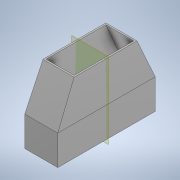
# Autodesk Inventor part: Guía
Saved by Autodesk Inventor 2020.3 (Build 243373000, 373)
## iProperties
Created: 2020-07-24
Part Number: Guía
Material: ABS Plastic
Document SubType Name: Modeling
Designer: juanp
Density: 1.06 g/cm^3
Appearance: Smooth - White
Author: juanp
Autodesk Inventor part; units mm, degrees
ref_plane "YZ Plane" through (0, 0, 0) normal (1, 0, 0) x (0, 1, 0)
ref_plane "XZ Plane" through (0, 0, 0) normal (0, 1, 0) x (-1, 0, 0)
ref_plane "XY Plane" through (0, 0, 0) normal (0, 0, 1) x (1, 0, 0)
sketch "Sketch1" plane through (0, 0, 0) normal (0, 1, 0) x (-1, 0, 0)
  line L0 (0, 0) -> (38, 0)
  line L1 (38, 0) -> (38, 120)
  line L2 (38, 120) -> (0, 120)
  line L3 (0, 120) -> (0, 0)
  line L4 (40, 122) -> (-2, 122)
  line L5 (-2, 122) -> (-2, -2)
  line L6 (-2, -2) -> (40, -2)
  line L7 (40, -2) -> (40, 122)
  line L8 (40, 122) -> (-2, -2) construction
  line L9 (-2, 122) -> (40, -2) construction
  line L10 (38, 120) -> (0, 0) construction
  line L11 (38, 0) -> (0, 120) construction
  point P0 (19, 60)
  point P1 (19, 60)
  dimension "d0" = 38
  dimension "d1" = 120
  dimension "d2" = 42
  dimension "d3" = 124
  constraints: 24 end point, 4 midpoint, 4 parallel, 2 horizontal, 2 perpendicular
  measures "d0" distance of L1.end L2.end
  measures "d1" distance of L0.end L1.end
  measures "d2" distance of L6.end L5.end
  measures "d3" distance of L5.end L4.end
extrude "Extrusion1" add sketch "Sketch1" along normal blind 38
ref_plane "Work Plane1" through (0, 88, 0) normal (0, 1, 0) x (1, 0, 0)
sketch "Sketch3" plane through (0, 38, 0) normal (0, 1, 0) x (1, 0, 0)
  line L0 (-40, 2) -> (-40, -122) projected
  line L1 (2, -122) -> (2, 2) projected
  line L2 (-40, 2) -> (2, 2)
  line L3 (2, 2) -> (2, -122)
  line L4 (2, -122) -> (-40, -122)
  line L5 (-40, -122) -> (-40, 2)
  line L6 (-38, -120) -> (-38, 0) projected
  line L7 (-38, -120) -> (0, -120)
  line L8 (0, -120) -> (0, 0)
  line L9 (0, 0) -> (-38, 0)
  line L10 (-38, 0) -> (-38, -120)
  constraints: 16 end point, 4 parallel, 2 horizontal, 2 perpendicular
sketch "Sketch2" plane through (0, 88, 0) normal (0, 1, 0) x (1, 0, 0)
  line L0 (-40, -122) -> (2, -122) projected
  line L1 (2, -122) -> (2, 2) projected
  line L2 (0, 0) -> (0, -120) projected
  line L3 (0, -120) -> (-38, -120) projected
  line L4 (-38, -120) -> (-38, 0) projected
  line L5 (-40, 2) -> (-40, -122) projected
  line L6 (-38, 0) -> (0, 0) projected
  line L7 (2, 2) -> (-40, 2) projected
  line L8 (-36.8, -98) -> (-1.2, -98)
  line L9 (-1.2, -98) -> (-1.2, -22)
  line L10 (-1.2, -22) -> (-36.8, -22)
  line L11 (-36.8, -22) -> (-36.8, -98)
  line L12 (-36.8, -98) -> (-1.2, -22) construction
  line L13 (-1.2, -98) -> (-36.8, -22) construction
  line L14 (-40, 2) -> (2, -122) construction
  line L15 (-40, -122) -> (2, 2) construction
  line L16 (-38.8, -100) -> (0.8, -100)
  line L17 (0.8, -100) -> (0.8, -20)
  line L18 (0.8, -20) -> (-38.8, -20)
  line L19 (-38.8, -20) -> (-38.8, -100)
  line L20 (-38.8, -100) -> (0.8, -20) construction
  line L21 (0.8, -100) -> (-38.8, -20) construction
  point P0 (-19, -60)
  point P1 (-19, -60)
  dimension "d7" = 35.6
  dimension "d8" = 76
  dimension "d9" = 39.6
  dimension "d10" = 80
  constraints: 28 end point, 6 midpoint, 4 parallel, 2 horizontal, 2 perpendicular
  measures "d7" distance of L10.end L9.end
  measures "d8" distance of L10.end L8.start
  measures "d9" distance of L18.end L17.end
  measures "d10" distance of L17.end L16.end
loft "Loft1" add profiles "Sketch3", "Sketch2" contours L2 L1 L4 L0 | L6 L9 L8 L7 / L18 L17 L16 L2 | L2 L16 L4 L18 | L4 L16 L19 L18 | L11 L10 L9 L8
loft "Loft2" cut profiles "Sketch2", "Sketch3" contours L11 L10 L9 L8 / L6 L9 L8 L7
ref_plane "Work Plane2" through (2, 0, 60) normal (0, 0, -1) x (-1, 0, 0)
body "Solid1"
